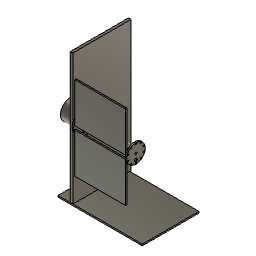
Flap-Display v11 (Autodesk Fusion 360 archive; units mm, degrees)
design "Flap-Display"
part number: Single Box Width
Autodesk Fusion 360 part; units mm, degrees
sketch "Skizze1" plane through (0, 0, 0) normal (0, 0, 1) x (1, 0, 0)
  line L0 (0, 0) -> (120, 0)
  line L1 (120, 0) -> (120, -80)
  line L2 (120, -80) -> (0, -80)
  line L3 (0, -80) -> (0, 0)
  line L4 (118, 0) -> (118, -78)
  line L5 (118, -78) -> (2, -78)
  line L6 (2, -78) -> (2, 0)
  dimension "d1" = 120
  dimension "d2" = 80
  dimension "d6" = 2
  constraint horizontal L0
  constraint vertical L1
  constraint horizontal L2
  constraint vertical L3
  constraint coincident L0.start L3.end
  measures "d1" distance of L0.start L0.end
  measures "d2" distance of L0.start L2.end
extrude "Extrusion3" add sketch "Skizze1" along normal blind 2 contours L0 L4 L5 L6 makes body 1
extrude "Extrusion4" add sketch "Skizze1" along normal blind 184 separate body contours L0 L1 L2 L3 L4 L5 L6 makes body 2
sketch "Skizze2" plane through (0, -80, 0) normal (0, -1, 0) x (1, 0, 0)
  line L0 (0, 0) -> (120, 0)
  line L1 (120, 0) -> (120, 184)
  line L2 (120, 184) -> (0, 184)
  line L3 (0, 184) -> (0, 0)
  line L4 (23, 184) -> (23, 0)
  line L5 (97, 0) -> (97, 184)
  line L6 (120, 149.5) -> (0, 149.5)
  line L7 (0, 34.5) -> (120, 34.5)
extrude "Extrusion5" cut sketch "Skizze2" against normal blind 2 contours L4 L5 L6 L7 bodies 2
sketch "Skizze9" plane through (0, -78, 0) normal (0, 1, 0) x (-1, 0, 0)
  line L0 (-97, 34.5) -> (-97, 149.5)
  line L1 (-23, 149.5) -> (-23, 34.5)
  line L2 (-118, 0) -> (-2, 0)
  line L3 (-2, 0) -> (-2, 184)
  line L4 (-2, 184) -> (-118, 184)
  line L5 (-118, 184) -> (-118, 0)
  line L6 (-23, 149.5) -> (-25, 149.5)
  line L7 (-25, 149.5) -> (-25, 151.5)
  line L8 (-25, 151.5) -> (-23, 151.5)
  line L9 (-23, 151.5) -> (-23, 149.5)
  line L10 (-25, 151.5) -> (-95, 151.5)
  line L11 (-95, 151.5) -> (-95, 96.5)
  line L12 (-95, 96.5) -> (-25, 96.5)
  line L13 (-25, 96.5) -> (-25, 151.5)
  line L14 (-25, 96.5) -> (-23, 96.5)
  line L15 (-23, 96.5) -> (-23, 91.5)
  line L16 (-23, 91.5) -> (-25, 91.5)
  line L17 (-25, 91.5) -> (-25, 96.5)
  line L18 (-25, 91.5) -> (-95, 91.5)
  line L19 (-95, 91.5) -> (-95, 36.5)
  line L20 (-95, 36.5) -> (-25, 36.5)
  line L21 (-25, 36.5) -> (-25, 91.5)
  line L22 (-23, 34.5) -> (-97, 34.5)
  line L23 (-97, 149.5) -> (-23, 149.5)
  dimension "d116" = 2
  dimension "d117" = 2
  dimension "d118" = 70
  dimension "d119" = 55
  dimension "d120" = 2
  dimension "d121" = 5
  dimension "d122" = 70
  dimension "d123" = 55
  constraint horizontal L6
  constraint vertical L7
  constraint horizontal L8
  constraint vertical L9
  constraint coincident L1.start L6.start
  constraint horizontal L10
  constraint vertical L11
  constraint horizontal L12
  constraint vertical L13
  constraint horizontal L14
  constraint vertical L15
  constraint horizontal L16
  constraint vertical L17
  constraint horizontal L18
  constraint vertical L19
  constraint horizontal L20
  constraint vertical L21
  measures "d116" distance of L1.start L6.end
  measures "d117" distance of L1.start L8.end
  measures "d118" distance of L7.end L10.end
  measures "d119" distance of L7.end L12.end
  measures "d120" distance of L12.end L14.end
  measures "d121" distance of L12.end L16.end
  measures "d122" distance of L16.end L18.end
  measures "d123" distance of L16.end L20.end
extrude "Extrusion20" add sketch "Skizze9" along normal blind 2 separate body contours L11 L12 L13 L23 | L7 L10 L11 L13 L23 makes body 3
extrude "Extrusion21" add sketch "Skizze9" along normal blind 2 separate body contours L18 L19 L20 L21 makes body 4
sketch "Skizze10" plane through (95, 0, 0) normal (1, 0, 0) x (0, 1, 0)
  line L0 (-78, 151.5) -> (-78, 96.5)
  line L1 (-78, 96.5) -> (-76, 96.5)
  line L2 (-76, 96.5) -> (-76, 151.5)
  line L3 (-76, 151.5) -> (-78, 151.5)
  line L4 (-78, 96.5) -> (-77, 96.5)
  line L5 (-77, 96.5) -> (-77, 97.5)
  line L6 (-77, 97.5) -> (-78, 97.5)
  line L7 (-78, 97.5) -> (-78, 96.5)
  circle A0 centre (-77, 97.5) radius 1
  line L8 (-78, 91.5) -> (-77, 91.5)
  line L9 (-77, 91.5) -> (-77, 90.5)
  line L10 (-77, 90.5) -> (-78, 90.5)
  line L11 (-78, 90.5) -> (-78, 91.5)
  circle A1 centre (-77, 90.5) radius 1
  point P0 (-78, 91.5)
  dimension "d128" = 1
  dimension "d129" = 1
  dimension "d130" = 2
  dimension "d131" = 1
  dimension "d132" = 1
  dimension "d133" = 2
  constraint horizontal L4
  constraint vertical L5
  constraint horizontal L6
  constraint vertical L7
  constraint coincident L0.end L1.start
  constraint coincident L5.end L6.start
  constraint horizontal L8
  constraint vertical L9
  constraint horizontal L10
  constraint vertical L11
  constraint coincident L9.end L10.start
  constraint coincident P0 L8.start
  measures "d128" distance of L0.end L4.end
  measures "d129" distance of L0.end L6.end
  measures "d130" diameter of A0
  measures "d131" distance of P0 L8.end
  measures "d132" distance of P0 L10.end
  measures "d133" diameter of A1
extrude "Extrusion22" add sketch "Skizze10" along normal blind 2.5 contours L5 L6 A0 | L5 L6 A0 | L9 L10 A1 | L9 L10 A1 bodies 3 4
sketch "Skizze11" plane through (25, 0, 0) normal (-1, 0, 0) x (0, -1, 0)
  line L0 (78, 96.5) -> (78, 151.5)
  line L1 (78, 151.5) -> (76, 151.5)
  line L2 (76, 151.5) -> (76, 96.5)
  line L3 (76, 96.5) -> (78, 96.5)
  line L4 (76, 96.5) -> (77, 96.5)
  line L5 (77, 96.5) -> (77, 97.5)
  line L6 (77, 97.5) -> (76, 97.5)
  line L7 (76, 97.5) -> (76, 96.5)
  line L8 (76, 91.5) -> (77, 91.5)
  line L9 (77, 91.5) -> (77, 90.5)
  line L10 (77, 90.5) -> (76, 90.5)
  line L11 (76, 90.5) -> (76, 91.5)
  circle A0 centre (77, 97.5) radius 1
  circle A1 centre (77, 90.5) radius 1
  point P0 (76, 91.5)
  dimension "d137" = 1
  dimension "d138" = 1
  dimension "d139" = 1
  dimension "d140" = 1
  dimension "d141" = 2
  dimension "d142" = 2
  constraint horizontal L4
  constraint vertical L5
  constraint horizontal L6
  constraint vertical L7
  constraint coincident L2.end L3.start
  constraint horizontal L8
  constraint vertical L9
  constraint horizontal L10
  constraint vertical L11
  constraint coincident L5.end L6.start
  constraint coincident L9.end L10.start
  constraint coincident P0 L8.start
  measures "d137" distance of L2.end L4.end
  measures "d138" distance of L2.end L6.end
  measures "d139" distance of P0 L8.end
  measures "d140" distance of P0 L10.end
  measures "d141" diameter of A0
  measures "d142" diameter of A1
extrude "Extrusion23" add sketch "Skizze11" along normal blind 2.5 contours L5 L6 A0 | L5 L6 A0 | L9 L10 A1 | L9 L10 A1 bodies 3 4
sketch "Skizze12" plane through (95, 0, 0) normal (1, 0, 0) x (0, 1, 0)
  arc A0 (-76, 97.5) -> (-78, 97.5) centre (-77, 97.5) ccw
  line L0 (-76, 97.5) -> (-76, 151.5)
  line L1 (-76, 151.5) -> (-78, 151.5)
  line L2 (-78, 151.5) -> (-78, 97.5)
  line L3 (-78, 95.1429) -> (-77, 95.1429)
  line L4 (-77, 95.1429) -> (-77, 92.6429)
  line L5 (-77, 92.6429) -> (-78, 92.6429)
  line L6 (-78, 92.6429) -> (-78, 95.1429)
  line L7 (-78, 91.5) -> (-77, 91.5)
  line L8 (-77, 91.5) -> (-77, 90.5)
  line L9 (-77, 90.5) -> (-78, 90.5)
  line L10 (-78, 90.5) -> (-78, 91.5)
  circle A1 centre (-77, 90.5) radius 1.05
  line L11 (-78, 91.5) -> (-66.2281, 91.5)
  line L12 (-66.2281, 91.5) -> (-66.2281, 94)
  line L13 (-66.2281, 94) -> (-78, 94)
  line L14 (-78, 94) -> (-78, 91.5)
  circle A2 centre (-72.8855, 84.8369) radius 1.05
  circle A3 centre (-66.2281, 82.6738) radius 1.05
  circle A4 centre (-59.5707, 84.8369) radius 1.05
  circle A5 centre (-55.4562, 90.5) radius 1.05
  circle A6 centre (-55.4562, 97.5) radius 1.05
  circle A7 centre (-59.5707, 103.1631) radius 1.05
  circle A8 centre (-66.2281, 105.3262) radius 1.05
  circle A9 centre (-72.8855, 103.1631) radius 1.05
  circle A10 centre (-77, 97.5) radius 1.05
  circle A11 centre (-66.2281, 94) radius 5.3859
  circle A12 centre (-66.2281, 94) radius 12.7719
  circle A13 centre (-66.2281, 86.1689) radius 2
  point P0 (-77, 92.6429)
  point P1 (-78, 91.5)
  point P2 (-66.2281, 86.1689)
  dimension "d145" = 1
  dimension "d146" = 2.5
  dimension "d149" = 1
  dimension "d150" = 1
  dimension "d151" = 2.1
  dimension "d155" = 11.7719
  dimension "d156" = 2.5
  dimension "d158" = 360
  dimension "d160" = 10.7719
  dimension "d163" = 25.5438
  dimension "d220" = 4
  constraint horizontal L3
  constraint vertical L4
  constraint horizontal L5
  constraint vertical L6
  constraint coincident P0 L4.end
  constraint horizontal L7
  constraint vertical L8
  constraint horizontal L9
  constraint vertical L10
  constraint coincident L8.end L9.start
  constraint coincident P1 L7.start
  constraint horizontal L11
  constraint vertical L12
  constraint horizontal L13
  constraint vertical L14
  constraint coincident L12.end L13.start
  constraint concentric A11 A12
  constraint coincident P2 A13.centre
  measures "d145" distance of L3.start L3.end
  measures "d146" distance of L3.start L5.end
  measures "d149" distance of P1 L7.end
  measures "d150" distance of P1 L9.end
  measures "d151" diameter of A1
  measures "d155" distance of P1 L11.end
  measures "d156" distance of P1 L13.end
  measures "d160" diameter of A11
  measures "d163" diameter of A12
  measures "d220" diameter of A13
extrude "Extrusion24" add sketch "Skizze12" along normal blind 2 separate body contours L0 L2 A10 A12 | L0 L2 A10 A12 | L3 L4 L6 L13 | L4 L5 L6 L13 L14 | L4 L5 L7 A1 L11 L13 L14 A11 | L11 L12 L13 A11 | L11 L12 L13 A11 | L7 L10 A1 L11 | A13 makes body 5
copy_body "Körper kopieren/einfügen1" bodies 5 makes body 6
move_body "Verschieben1" bodies 6 to x (1, 0, 0) y (0, 1, 0) z (0, 0, 1) at (-72, 0, 0)
move_body "Verschieben2" bodies 6 to x (1, 0, 0) y (0, 1, 0) z (0, 0, 1) at (-0.5, 0, 0)
move_body "Verschieben3" bodies 5 to x (1, 0, 0) y (0, 1, 0) z (0, 0, 1) at (0.5, 0, 0)
sketch "Skizze13" plane through (22.5, 0, 0) normal (-1, 0, 0) x (0, -1, 0)
  circle A0 centre (72.8855, 84.8369) radius 1.05
  circle A1 centre (66.2281, 105.3262) radius 1.05
  circle A2 centre (66.2281, 82.6738) radius 1.05
  circle A3 centre (55.4562, 90.5) radius 1.05
  circle A4 centre (77, 90.5) radius 1.05
  circle A5 centre (59.5707, 84.8369) radius 1.05
  circle A6 centre (59.5707, 103.1631) radius 1.05
  circle A7 centre (77, 97.5) radius 1.05
  circle A8 centre (55.4562, 97.5) radius 1.05
  circle A9 centre (72.8855, 103.1631) radius 1.05
  circle A10 centre (66.2281, 94) radius 12.7719
  line L0 (78, 2) -> (-2, 2)
  line L1 (-2, 2) -> (-2, 182)
  line L2 (-2, 182) -> (78, 182)
  line L3 (78, 182) -> (78, 2)
  circle A11 centre (66.2281, 94) radius 2.5
  circle A12 centre (66.2281, 94) radius 4.6
  line L4 (70.8281, 94) -> (72.2581, 94)
  line L5 (72.2581, 94) -> (58.2581, 94)
  circle A13 centre (58.2581, 94) radius 14
  circle A14 centre (58.2581, 94) radius 20.95
  line L6 (58.2581, 108) -> (58.2581, 114.95)
  circle A15 centre (58.2581, 111.475) radius 1.9
  circle A16 centre (58.2581, 111.475) radius 3.475
  line L7 (54.7831, 116) -> (54.7831, 70)
  line L8 (61.7331, 116) -> (61.7331, 70)
  line L9 (58.2581, 80) -> (58.2581, 73.05)
  circle A17 centre (58.2581, 76.525) radius 1.9
  circle A18 centre (58.2581, 76.525) radius 3.475
  line L10 (66.2281, 94) -> (67.6781, 94)
  line L11 (66.2281, 94) -> (64.7781, 94)
  line L12 (67.6781, 94) -> (67.6781, 91.7)
  line L13 (67.6781, 94) -> (67.6781, 96.3397)
  line L14 (64.7781, 94) -> (64.7781, 96.2178)
  line L15 (64.7781, 94) -> (64.7781, 91.7259)
  point P0 (66.2281, 94)
  point P1 (58.2581, 111.475)
  point P2 (58.2581, 76.525)
  dimension "d168" = 80
  dimension "d169" = 180
  dimension "d178" = 5
  dimension "d179" = 9.2
  dimension "d182" = 1.43
  dimension "d183" = 14
  dimension "d184" = 28
  dimension "d185" = 41.9
  dimension "d187" = 3.8
  dimension "d188" = 3.8
  dimension "d190" = 1.45
  dimension "d191" = 1.45
  constraint coincident P0 A10.centre
  constraint horizontal L0
  constraint vertical L1
  constraint horizontal L2
  constraint vertical L3
  constraint coincident A12 L4.start
  constraint parallel L4 L5
  constraint coincident L5.end A13.centre
  constraint concentric A13 A14
  constraint coincident A14 L6.end
  constraint coincident A13 L6.start
  constraint midpoint L6 P1
  constraint coincident P1 A15.centre
  constraint coincident L6.end A16
  constraint vertical L7
  constraint vertical L8
  constraint tangent A16 L7
  constraint tangent A16 L8
  constraint coincident A14 L9.end
  constraint coincident A13 L9.start
  constraint midpoint P2 L9
  constraint coincident P2 A17.centre
  constraint coincident L9.end A18
  constraint tangent A14 A18
  constraint perpendicular L8 L10
  constraint parallel L5 L11
  constraint perpendicular L10 L12
  constraint perpendicular L10 L13
  constraint perpendicular L11 L14
  constraint perpendicular L11 L15
  measures "d168" distance of L0.start L0.end
  measures "d169" distance of L0.start L2.end
  measures "d178" diameter of A11
  measures "d179" diameter of A12
  measures "d182" distance of L4.start L4.end
  measures "d183" distance of L4.end L5.end
  measures "d184" diameter of A13
  measures "d185" diameter of A14
  measures "d187" diameter of A15
  measures "d188" diameter of A17
  measures "d190" distance of P0 L10.end
  measures "d191" distance of P0 L11.end
extrude "Extrusion25" add sketch "Skizze13" along normal blind 19.4 separate body contours A1 A13 | A1 A10 A12 L4 L5 A13 L8 | A10 A13 L8 | A2 A10 A12 L4 L5 A13 L8 | A3 A8 A10 A12 L7 L8 | A10 A13 L7 L8 | A11 A12 L5 L8 | A11 A12 L5 L8 | A2 A13 | A3 A8 A10 L7 | A10 A13 L7 | A12 L5 L8 | A12 L5 L8 | A11 L5 L13 | A11 L5 L12 | A10 A13 L7 L8 | A8 L7 | A8 L7 | A10 A13 L8 | A11 L5 L10 L11 L13 L14 | A11 L5 L10 L11 L12 L15 | A3 L7 | A3 L7 | A11 L5 L15 | A11 L5 L14 | A5 | A6 picked at (66.1042, 105.1059) picked at (66.1042, 82.8941) makes body 7
extrude "Extrusion26" add sketch "Skizze13" along normal blind 0.85 contours A13 A16 L8 | L6 A15 A16 | L6 A15 A16 | A13 A16 L7 | A13 L7 A18 | A13 L8 A18 | L9 A17 A18 | L9 A17 A18 bodies 7
extrude "Extrusion27" add sketch "Skizze13" against normal blind 1.5 contours A11 A12 L5 L8 | A11 A12 L5 L8 | A11 L5 L13 | A11 L5 L12 | A11 L5 L10 L11 L13 L14 | A11 L5 L10 L11 L12 L15 | A11 L5 L15 | A11 L5 L14 bodies 7
extrude "Extrusion28" add sketch "Skizze13" against normal blind 2 from surface at -1.5 separate body contours A11 L5 L13 | A11 L5 L12 | A11 L5 L10 L11 L13 L14 | A11 L5 L10 L11 L12 L15 | A11 L5 L15 | A11 L5 L14 makes body 8
extrude "Extrusion29" add sketch "Skizze13" against normal blind 6 from surface at -3.5 separate body contours A11 L5 L10 L11 L13 L14 | A11 L5 L10 L11 L12 L15 makes body 9
combine "Kombinieren1" operation add target body 8 tool bodies 9
combine "Kombinieren2" operation add target body 7 tool bodies 8
extrude "Extrusion30" cut sketch "Skizze13" against normal blind 2 contours A11 L5 L10 L11 L13 L14 | A11 L5 L10 L11 L12 L15 bodies 6
move_body "Verschieben4" bodies 7 to x (1, 0, 0) y (0, 1, 0) z (0, 0, 1) at (-3.5, 0, 0)
extrude "Extrusion33" add sketch "Skizze13" along normal blind 3.5 separate body contours A0 | A1 A13 | A1 A2 A4 A7 A10 L3 A13 | A1 A13 | A1 A10 A12 L4 L5 A13 L8 | A10 L3 A13 A14 L8 | A10 A13 L8 | A2 A10 A12 L4 L5 A13 L8 | A3 A8 A10 A12 L7 L8 | A10 A13 L7 L8 | A13 A16 L8 | A11 A12 L5 L8 | A11 A12 L5 L8 | A2 A13 | A2 A13 | L0 L1 L2 L3 A14 | A7 L3 | A3 A8 A10 L7 | A10 A13 L7 | A12 L5 L8 | L6 A15 A16 | L6 A15 A16 | A13 A16 L7 | A14 A16 L8 | A12 L5 L8 | A11 L5 L13 | A11 L5 L12 | A10 L3 A13 A14 L8 | A10 A13 L7 L8 | A13 A14 L7 | A8 L7 | A8 L7 | L6 A15 | L6 A15 | A14 A16 L7 | A10 A13 L8 | A11 L5 L10 L11 L13 L14 | A11 L5 L10 L11 L12 L15 | A4 L3 | A3 L7 | A3 L7 | A13 L7 A18 | A11 L5 L15 | A11 L5 L14 | A13 L8 A18 | A14 L8 A18 | L9 A17 A18 | L9 A17 A18 | A14 L7 A18 | L9 A17 | L9 A17 | A5 | A6 | A9 picked at (77.3321, 97.3972) picked at (77.2971, 90.4517) makes body 10
extrude "Extrusion34" cut sketch "Skizze13" along normal blind 3.5 contours A11 A12 L5 L8 | A11 A12 L5 L8 | A12 L5 L8 | A12 L5 L8 | A11 L5 L13 | A11 L5 L12 | A11 L5 L10 L11 L13 L14 | A11 L5 L10 L11 L12 L15 | A11 L5 L15 | A11 L5 L14 bodies 10
extrude "Extrusion35" cut sketch "Skizze13" along normal blind 3.5 contours L6 A15 | L6 A15 | L9 A17 | L9 A17 bodies 10
thread "Gewinde1" "ISO Metric profile 3.5 M3.5x0.6 6H" major diameter 3.5995 minor diameter 2.93 pitch 0.6 angle 60 resizes the face on face at (20.1667, -60.1487, 111.6642) on bodies 10
thread "Gewinde2" "ISO Metric profile 3.5 M3.5x0.6 6H" major diameter 3.5995 minor diameter 2.93 pitch 0.6 angle 60 resizes the face on face at (20.1667, -59.5848, 77.8851) on bodies 10
extrude "Extrusion36" add sketch "Skizze12" against normal blind 1 separate body contours A13 makes body 11
move_body "Verschieben5" bodies 11 to x (1, 0, 0) y (0, 1, 0) z (0, 0, 1) at (2.5, 0, 0)
extrude "Extrusion37" cut 1 faces at (97.5, -66.7168, 85.5167) along direction (-1, 0, 0) blind 1 on bodies 11 bodies 5 11
extrude "Extrusion38" cut sketch "Skizze12" against normal blind 72 contours L11 L12 L13 A11 | L11 L12 L13 A11 bodies 6
extrude "Extrusion39" add sketch "Skizze12" against normal blind 71 separate body contours L11 L12 L13 A11 | L11 L12 L13 A11 makes body 12
extrude "Extrusion40" add sketch "Skizze12" along normal blind 0.5 separate body contours L11 L12 L13 A11 | L11 L12 L13 A11 makes body 13
combine "Kombinieren3" operation add target body 12 tool bodies 13
extrude "Extrusion41" add 1 faces at (23, -68.9901, 94) along direction (1, 0, 0) blind 1.5 on bodies 6 bodies 6 11
extrude "Extrusion42" cut sketch "Skizze13" against normal blind 7 contours A11 L5 L10 L11 L13 L14 | A11 L5 L10 L11 L12 L15 bodies 12
sketch "Skizze15" plane through (97.5, 0, 0) normal (1, 0, 0) x (0, 1, 0)
  circle A0 centre (-66.2281, 86.1689) radius 2
  circle A1 centre (-59.5707, 103.1631) radius 1.05
  circle A2 centre (-77, 97.5) radius 1.05
  circle A3 centre (-66.2281, 105.3262) radius 1.05
  circle A4 centre (-55.4562, 90.5) radius 1.05
  circle A5 centre (-55.4562, 97.5) radius 1.05
  circle A6 centre (-59.5707, 84.8369) radius 1.05
  circle A7 centre (-66.2281, 82.6738) radius 1.05
  circle A8 centre (-72.8855, 84.8369) radius 1.05
  circle A9 centre (-72.8855, 103.1631) radius 1.05
  circle A10 centre (-77, 90.5) radius 1.05
  circle A11 centre (-66.2281, 94) radius 12.7719
  circle A12 centre (-66.2281, 94) radius 1.5
  circle A13 centre (-66.2281, 94) radius 4
  point P0 (-66.2281, 94)
  dimension "d236" = 3
  dimension "d237" = 8
  constraint coincident P0 A11.centre
  constraint concentric A12 A13
  measures "d236" diameter of A12
  measures "d237" diameter of A13
extrude "Extrusion43" cut sketch "Skizze15" against normal blind 2 contours A12 bodies 5
extrude "Extrusion10" [suppressed]
delete_face "Fläche löschen1" [suppressed]
extrude "Extrusion17" [suppressed]
extrude "Extrusion18" [suppressed]
extrude "Extrusion19" [suppressed]
hidden bodies 2
equation "d1 = SingleFlapBox_Breite"
equation "d2 = SingleFlapBox_Tiefe"
equation "SingleFlapBox_Breite = 120 mm"
equation "SingleFlapBox_Tiefe = 80 mm"
equation "SingleFlapBox_InnereHöhe = 180 mm"
equation "d6 = SingleFlapBox_Wandstärke"
equation "SingleFlapBox_Wandstärke = 2 mm"
equation "SingleFlapBox_ÄußereHöhe = SingleFlapBox_InnereHöhe + 2 * SingleFlapBox_Wandstärke"
equation "d13 = SingleFlapBox_Wandstärke"
equation "d15 = SingleFlapBox_ÄußereHöhe"
equation "SingleFlapBox_Rahmen_Horizontal = ( SingleFlapBox_Breite - Flap_Breite - Flap_Zwischenraum_Links - Flap_Zwischenraum_Rechts ) / 2"
equation "SingleFlapBox_Rahmen_Vertikal = ( SingleFlapBox_ÄußereHöhe - 2 * Flap_Höhe + Flap_Zwischenraum_Oben - Flap_Zwischenraum_Unten - Flap_ZwischenraumZwischenFlaps ) / 2"
equation "Flap_Breite = 70 mm"
equation "Flap_Höhe = 55 mm"
equation "d21 = -SingleFlapBox_Rahmen_Horizontal"
equation "d22 = -SingleFlapBox_Rahmen_Horizontal"
equation "d23 = -SingleFlapBox_Rahmen_Vertikal"
equation "d24 = -SingleFlapBox_Rahmen_Vertikal"
equation "d25 = -SingleFlapBox_Wandstärke"
equation "Flap_Zwischenraum_Links = 2 mm"
equation "Flap_Zwischenraum_Rechts = 2 mm"
equation "Flap_Zwischenraum_Oben = 2 mm"
equation "Flap_Zwischenraum_Unten = 2 mm"
equation "Flap_ZwischenraumZwischenFlaps = 5 mm"
equation "Flap_Tiefe = 2 mm"
equation "d53 = Flap_Tiefe"
equation "Flap_Abrundung = 1 mm"
equation "FlapHalter_Dicke = 2 mm"
equation "FlapHalter_AbstandZuFlaps = 1 mm"
equation "FlapHalter_AnzahlFlaps = 10"
equation "FlapHalter_RadiusZuPunktZwischenZweiFlaps = ( FlapHalter_MittelpunktZwischenFlaps / tan(( 360 / ( 2 * FlapHalter_AnzahlFlaps ) ) * 1 deg) )"
equation "Flap_NubsiDurchmesser = Flap_Tiefe"
equation "SingleFlapBox_Ausschnitt_Breite = Flap_Breite + Flap_Zwischenraum_Links + Flap_Zwischenraum_Rechts"
equation "SingleFlapBox_Ausschnitt_Höhe = Flap_Höhe + Flap_Zwischenraum_Oben + Flap_Zwischenraum_Unten"
equation "d110 = -Flap_Tiefe"
equation "d112 = Flap_Tiefe"
equation "d114 = Flap_Tiefe"
equation "d116 = Flap_Zwischenraum_Links"
equation "d117 = Flap_Zwischenraum_Oben"
equation "d118 = Flap_Breite"
equation "d119 = Flap_Höhe"
equation "d120 = Flap_Zwischenraum_Links"
equation "d121 = Flap_ZwischenraumZwischenFlaps"
equation "d122 = Flap_Breite"
equation "d123 = Flap_Höhe"
equation "d124 = Flap_Tiefe"
equation "d126 = Flap_Tiefe"
equation "d128 = Flap_NubsiDurchmesser / 2"
equation "d129 = Flap_NubsiDurchmesser / 2"
equation "d130 = Flap_NubsiDurchmesser"
equation "d131 = Flap_NubsiDurchmesser / 2"
equation "d132 = Flap_NubsiDurchmesser / 2"
equation "d133 = Flap_NubsiDurchmesser"
equation "Flap_Nubsi_Tiefe = FlapHalter_Dicke + FlapHalter_zu_Flap_Spielraum"
equation "d135 = Flap_Nubsi_Tiefe"
equation "d137 = Flap_NubsiDurchmesser / 2"
equation "d138 = Flap_NubsiDurchmesser / 2"
equation "d139 = Flap_NubsiDurchmesser / 2"
equation "d140 = Flap_NubsiDurchmesser / 2"
equation "d141 = Flap_NubsiDurchmesser"
equation "d142 = Flap_NubsiDurchmesser"
equation "d143 = Flap_Nubsi_Tiefe"
equation "d145 = Flap_NubsiDurchmesser / 2"
equation "d146 = Flap_ZwischenraumZwischenFlaps / 2"
equation "FlapHalter_MittelpunktZwischenFlaps = Flap_NubsiDurchmesser / 2 + Flap_ZwischenraumZwischenFlaps / 2"
equation "d149 = Flap_NubsiDurchmesser / 2"
equation "d150 = Flap_NubsiDurchmesser / 2"
equation "d151 = Flap_NubsiDurchmesser + FlapHalter_Loch_Spielraum"
equation "d155 = FlapHalter_Mittelpunkt_bis_FlapAußen"
equation "d156 = Flap_ZwischenraumZwischenFlaps / 2"
equation "d157 = FlapHalter_AnzahlFlaps"
equation "FlapHalter_Sphäre_Durchmesser = FlapHalter_RadiusZuPunktZwischenZweiFlaps"
equation "d160 = FlapHalter_Sphäre_Durchmesser"
equation "FlapHalter_Radius_Außen = FlapHalter_Mittelpunkt_bis_FlapAußen + Flap_NubsiDurchmesser / 2"
equation "FlapHalter_Mittelpunkt_bis_FlapAußen = Flap_NubsiDurchmesser / 2 + FlapHalter_RadiusZuPunktZwischenZweiFlaps"
equation "d163 = FlapHalter_Radius_Außen * 2"
equation "FlapHalter_Loch_Spielraum = 0.1 mm"
equation "d165 = FlapHalter_Dicke"
equation "FlapHalter_zu_Flap_Spielraum = 0.5 mm"
equation "d168 = SingleFlapBox_Tiefe"
equation "d169 = SingleFlapBox_InnereHöhe"
equation "Motor_Durchmesser = 28 mm"
equation "Motor_Tiefe = 19.40 mm"
equation "Motor_Durchmesser_Inkl_Befestigung = 41.9 mm"
equation "Motor_Vertiefung = 1.5 mm"
equation "Motor_Antrieb_Gesamt = 8 mm"
equation "Motor_Antrieb_Gefeilt = 6 mm"
equation "Motor_Vertiefung_Durchmesser = 9.2 mm"
equation "Motor_Antrieb_Durchmesser = 5 mm"
equation "d178 = Motor_Antrieb_Durchmesser"
equation "d179 = Motor_Vertiefung_Durchmesser"
equation "Motor_Abstand_Umfang_Vertiefung = 1.43 mm"
equation "d182 = Motor_Abstand_Umfang_Vertiefung"
equation "d183 = Motor_Durchmesser / 2"
equation "d184 = Motor_Durchmesser"
equation "d185 = Motor_Durchmesser_Inkl_Befestigung"
equation "Motor_Befestigung_Loch_Durchmesser = 3.8 mm"
equation "d187 = Motor_Befestigung_Loch_Durchmesser"
equation "d188 = Motor_Befestigung_Loch_Durchmesser"
equation "Motor_Antrieb_Breite = 2.9 mm"
equation "d190 = Motor_Antrieb_Breite / 2"
equation "d191 = Motor_Antrieb_Breite / 2"
equation "d192 = Motor_Tiefe"
equation "Motor_Befestigung_Tiefe = 0.85 mm"
equation "d195 = Motor_Befestigung_Tiefe"
equation "d197 = -Motor_Vertiefung"
equation "d199 = -Motor_Vertiefung"
equation "d200 = -( Motor_Antrieb_Gesamt - Motor_Antrieb_Gefeilt )"
equation "d202 = -( Motor_Vertiefung + Motor_Antrieb_Gesamt - Motor_Antrieb_Gefeilt )"
equation "d203 = -Motor_Antrieb_Gefeilt"
equation "d205 = -FlapHalter_Dicke"
equation "Komponentenhalter_Dicke = Motor_Vertiefung + ( Motor_Antrieb_Gesamt - Motor_Antrieb_Gefeilt )"
equation "d212 = Komponentenhalter_Dicke"
equation "d214 = Komponentenhalter_Dicke"
equation "d216 = Komponentenhalter_Dicke"
equation "Magnet_Durchmesser = 4 mm"
equation "Magnet_Tiefe = 1 mm"
equation "d220 = Magnet_Durchmesser"
equation "d221 = -Magnet_Tiefe"
equation "d223 = -Magnet_Tiefe"
equation "FlapHalter_Achse_Durchmesser = 10 mm"
equation "d226 = -( Flap_Breite + 2 * FlapHalter_AbstandZuFlaps )"
equation "d228 = -( Flap_Breite + FlapHalter_AbstandZuFlaps )"
equation "d230 = FlapHalter_AbstandZuFlaps / 2"
equation "d232 = FlapHalter_AbstandZuFlaps + FlapHalter_AbstandZuFlaps / 2"
equation "d234 = -( FlapHalter_Dicke + 5 mm )"
equation "d238 = -FlapHalter_Dicke"
named bodies: "Boden", "Wand", "Flap Oben", "Flap Unten", "Flaphalter Rechts", "Flaphalter Links", "Motor", "Rotations-Nubsi", "Komponentenhalter", "Magnet", "Achse"
